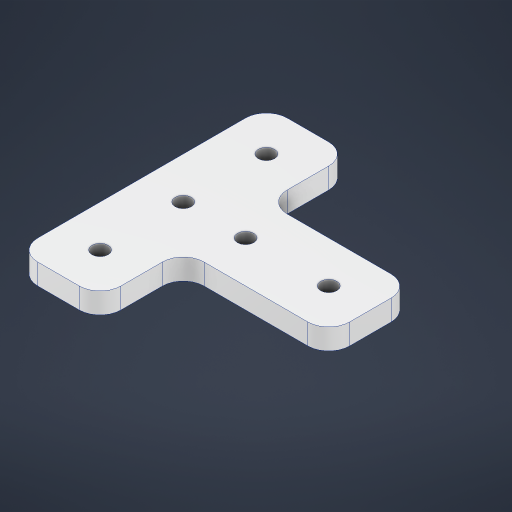
# Autodesk Inventor part: STRU_022_DVBSBracket3
Saved by Autodesk Inventor 2024.2 (Build 282272000, 272)
## iProperties
Created: 2024-07-28
Part Number: STRU_022_DVBSBracket3
Material: Aluminum 6061
Document SubType Name: Modeling
Designer: Bryan
Density: 2.7 g/cm^3
Appearance: Aluminum - Flat
Author: Bryan
Autodesk Inventor part; units mm, degrees
ref_plane "YZ Plane" through (0, 0, 0) normal (1, 0, 0) x (0, 1, 0)
ref_plane "XZ Plane" through (0, 0, 0) normal (0, 1, 0) x (-1, 0, 0)
ref_plane "XY Plane" through (0, 0, 0) normal (0, 0, 1) x (1, 0, 0)
sketch "Sketch1" plane through (0, 0, 0) normal (0, 1, 0) x (-1, 0, 0)
  circle A0 centre (0, 0) radius 2.4892
  circle A1 centre (0, 25.4) radius 2.4892
  circle A2 centre (0, -25.4) radius 2.4892
  circle A3 centre (-19.05, 0) radius 2.4892
  circle A4 centre (-44.45, 0) radius 2.4892
  line L0 (12.7, 38.1) -> (-12.7, 38.1)
  line L1 (-12.7, 38.1) -> (-12.7, 12.7)
  line L2 (-12.7, 12.7) -> (-57.15, 12.7)
  line L3 (-57.15, 12.7) -> (-57.15, -12.7)
  line L4 (-57.15, -12.7) -> (-12.7, -12.7)
  line L5 (-12.7, -12.7) -> (-12.7, -38.1)
  line L6 (-12.7, -38.1) -> (12.7, -38.1)
  line L7 (12.7, -38.1) -> (12.7, 38.1)
  point P0 (-57.15, 0)
  point P1 (0, 38.1)
  dimension "d0" = 4.9784
  dimension "d1" = 25.4
  dimension "d2" = 25.4
  dimension "d3" = 19.05
  dimension "d4" = 25.4
  dimension "d5" = 25.4
  dimension "d6" = 12.7
  dimension "d7" = 12.7
  dimension "d8" = 12.7
  constraints: 16 end point, 7 perpendicular, 5 centre point, 4 equal radius, 3 horizontal alignment, 3 vertical alignment, 2 equal length, 2 midpoint, 1 coincident, 1 horizontal
  measures "d0" diameter of A0
  measures "d1" distance of point (0, 0) A1.centre
  measures "d2" distance of A2.centre point (0, 0)
  measures "d3" distance of A3.centre point (0, 0)
  measures "d4" distance of A3.centre A4.centre
  measures "d5" distance of L0.start L0.end
  measures "d6" distance from line of L6 A2.centre
  measures "d7" distance from line of A1.centre L0
  measures "d8" distance from line of A4.centre L3
extrude "Extrusion1" add sketch "Sketch1" along normal blind 6.35
fillet "Fillet1" radius 6.35 8 edges at (-12.7, 3.175, 38.1) (12.7, 3.175, 38.1) (12.7, 3.175, 12.7) (57.15, 3.175, 12.7) (57.15, 3.175, -12.7) (12.7, 3.175, -12.7) (12.7, 3.175, -38.1) (-12.7, 3.175, -38.1)
body "Solid1"
